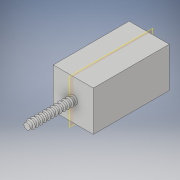
# Autodesk Inventor part: Square-Circle-Adapter V1D2-OUT
Saved by Autodesk Inventor 2017 (Build 210142000, 142)
## iProperties
Created: 2017-12-22
Part Number: Square-Circle-Adapter V1D2-OUT
Material: Generic
Document SubType Name: Modeling
Designer: Tripl_000
Density: 1 g/cm^3
Appearance: Default
Author: Tripl_000
Autodesk Inventor part; units mm, degrees
ref_plane "YZ Plane" through (0, 0, 0) normal (1, 0, 0) x (0, 1, 0)
ref_plane "XZ Plane" through (0, 0, 0) normal (0, 1, 0) x (-1, 0, 0)
ref_plane "XY Plane" through (0, 0, 0) normal (0, 0, 1) x (1, 0, 0)
sketch "Sketch1" plane through (0, 0, 0) normal (0, 0, 1) x (1, 0, 0)
  line L0 (-6.604, 6.604) -> (6.604, 6.604)
  line L1 (6.604, 6.604) -> (6.604, -6.604)
  line L2 (6.604, -6.604) -> (-6.604, -6.604)
  line L3 (-6.604, -6.604) -> (-6.604, 6.604)
  line L4 (-6.604, 6.604) -> (6.604, -6.604) construction
  line L5 (6.604, 6.604) -> (-6.604, -6.604) construction
  point P0 (0, 0)
  dimension "d0" = 13.208
  dimension "d1" = 13.208
  constraints: 12 end point, 2 midpoint, 2 parallel, 1 horizontal, 1 perpendicular
  measures "d0" distance of L2.end L0.start
  measures "d1" distance of L0.start L0.end
extrude "Extrusion1" add sketch "Sketch1" along normal blind 15
sketch "Sketch2" plane through (0, 0, 15) normal (0, 0, 1) x (1, 0, 0)
  line L0 (-5.0165, 5.0165) -> (5.0165, 5.0165)
  line L1 (5.0165, 5.0165) -> (5.0165, -5.0165)
  line L2 (5.0165, -5.0165) -> (-5.0165, -5.0165)
  line L3 (-5.0165, -5.0165) -> (-5.0165, 5.0165)
  line L4 (-5.0165, 5.0165) -> (5.0165, -5.0165) construction
  line L5 (5.0165, 5.0165) -> (-5.0165, -5.0165) construction
  point P0 (0, 0)
  dimension "d4" = 10.033
  dimension "d5" = 10.033
  constraints: 12 end point, 2 midpoint, 2 parallel, 1 horizontal, 1 perpendicular
  measures "d4" distance of L0.end L1.end
  measures "d5" distance of L0.start L0.end
extrude "Extrusion2" cut sketch "Sketch2" against normal through all
sketch "Sketch5" plane through (0, 0, 15) normal (0, 0, 1) x (1, 0, 0)
  line L0 (6.604, 6.604) -> (-6.604, 6.604) projected
  line L1 (6.604, 6.604) -> (6.604, -6.604) projected
  line L2 (-6.604, 6.604) -> (6.604, 6.604)
  line L3 (6.604, 6.604) -> (6.604, -6.604)
  line L4 (6.604, -6.604) -> (-6.604, -6.604)
  line L5 (-6.604, -6.604) -> (-6.604, 6.604)
  point P0 (0, 0)
  constraints: 8 end point, 2 parallel, 1 horizontal, 1 perpendicular
extrude "Extrusion5" add sketch "Sketch5" along normal blind 10
sketch "Sketch8" plane through (0, 0, 25) normal (0, 0, 1) x (1, 0, 0)
  circle A0 centre (0, 0) radius 0.762
  dimension "d44" = 1.524
  constraints: 1 centre point, 1 coincident
  measures "d44" diameter of A0
extrude "Extrusion7" add sketch "Sketch8" along normal blind 15.24
sketch "Sketch9" plane through (0, 0, 25) normal (0, 0, 1) x (1, 0, 0)
  circle A0 centre (0, 0) radius 1.016
  dimension "d47" = 2.032
  constraints: 1 centre point, 1 coincident
  measures "d47" diameter of A0
extrude "Extrusion8" add sketch "Sketch9" along normal up to surface (15.24 mm away)
ref_plane "Work Plane3" through (0, -6.604, 0) normal (1, 0, 0) x (0, 0, -1)
sketch "Sketch10" plane through (0, -6.604, 0) normal (1, 0, 0) x (0, 0, -1)
  line L0 (21.7384, 6.604) -> (-63.7893, 6.604)
  line L1 (-25, 5.588) -> (-25, 7.62) projected
  line L2 (-25, 7.62) -> (-25, 8.001)
  line L3 (-25, 0) -> (-25, 13.208) projected
  line L4 (-25, 8.001) -> (-25.381, 7.62)
  line L5 (-25, 7.62) -> (-40.24, 7.62) projected
  line L6 (-25.381, 7.62) -> (-25, 7.62)
  line L7 (-26.27, 7.62) -> (-26.27, 8.001)
  line L8 (-26.27, 8.001) -> (-26.651, 7.62)
  line L9 (-26.651, 7.62) -> (-26.27, 7.62)
  line L10 (-27.54, 7.62) -> (-27.54, 8.001)
  line L11 (-27.54, 8.001) -> (-27.921, 7.62)
  line L12 (-28.81, 7.62) -> (-28.81, 8.001)
  line L13 (-28.81, 8.001) -> (-29.191, 7.62)
  line L14 (-29.191, 7.62) -> (-28.81, 7.62)
  line L15 (-30.08, 7.62) -> (-30.08, 8.001)
  line L16 (-30.08, 8.001) -> (-30.461, 7.62)
  line L17 (-30.08, 7.62) -> (-30.461, 7.62)
  line L18 (-31.35, 7.62) -> (-31.35, 8.001)
  line L19 (-31.35, 8.001) -> (-31.731, 7.62)
  line L20 (-31.731, 7.62) -> (-31.35, 7.62)
  line L21 (-32.62, 7.62) -> (-32.62, 8.001)
  line L22 (-32.62, 8.001) -> (-33.001, 7.62)
  line L23 (-32.62, 7.62) -> (-33.001, 7.62)
  line L24 (-33.89, 7.62) -> (-33.89, 8.001)
  line L25 (-33.89, 8.001) -> (-34.271, 7.62)
  line L26 (-33.89, 7.62) -> (-34.271, 7.62)
  line L27 (-35.16, 7.62) -> (-35.16, 8.001)
  line L28 (-35.16, 8.001) -> (-35.541, 7.62)
  line L29 (-35.16, 7.62) -> (-35.541, 7.62)
  line L30 (-36.43, 7.62) -> (-36.43, 8.001)
  line L31 (-36.43, 8.001) -> (-36.811, 7.62)
  line L32 (-36.43, 7.62) -> (-36.811, 7.62)
  line L33 (-37.7, 7.62) -> (-37.7, 8.001)
  line L34 (-37.7, 8.001) -> (-38.081, 7.62)
  line L35 (-37.7, 7.62) -> (-38.081, 7.62)
  line L36 (-38.97, 7.62) -> (-38.97, 8.001)
  line L37 (-38.97, 8.001) -> (-39.351, 7.62)
  line L38 (-38.97, 7.62) -> (-39.351, 7.62)
  line L39 (-27.921, 7.62) -> (-27.54, 7.62)
  point P0 (0, 6.604)
  dimension "d51" = 0.381
  dimension "d52" = 45
  dimension "d53" = 0.381
  dimension "d54" = 0.381
  dimension "d55" = 0.381
  dimension "d56" = 0.381
  dimension "d57" = 0.381
  dimension "d58" = 0.381
  dimension "d59" = 0.381
  dimension "d60" = 0.381
  dimension "d61" = 0.381
  dimension "d62" = 0.381
  dimension "d63" = 0.381
  dimension "d64" = 1.27
  dimension "d65" = 1.27
  dimension "d66" = 1.27
  dimension "d67" = 1.27
  dimension "d68" = 1.27
  dimension "d69" = 1.27
  dimension "d70" = 1.27
  dimension "d71" = 1.27
  dimension "d72" = 1.27
  dimension "d73" = 1.27
  dimension "d74" = 1.27
  dimension "d75" = 0.381
  dimension "d76" = 0.381
  constraints: 74 end point, 11 vertical, 9 horizontal, 9 parallel, 4 perpendicular, 1 point on line, 23 other
  measures "d51" distance of L1.end L2.end
  measures "d52" angle of L2 L4
  measures "d53" distance of L36.start L36.end
  measures "d54" distance of L33.start L33.end
  measures "d55" distance of L30.start L30.end
  measures "d56" distance of L27.start L27.end
  measures "d57" distance of L24.start L24.end
  measures "d58" distance of L21.start L21.end
  measures "d59" distance of L18.start L18.end
  measures "d60" distance of L15.start L15.end
  measures "d61" distance of L12.start L12.end
  measures "d62" distance of L10.start L10.end
  measures "d63" distance of L7.start L7.end
  measures "d64" distance between parallel lines of L33 L36
  measures "d65" distance between parallel lines of L30 L33
  measures "d66" distance between parallel lines of L27 L30
  measures "d67" distance between parallel lines of L24 L27
  measures "d68" distance between parallel lines of L21 L24
  measures "d69" distance between parallel lines of L18 L21
  measures "d70" distance between parallel lines of L15 L18
  measures "d71" distance between parallel lines of L12 L15
  measures "d72" distance between parallel lines of L10 L12
  measures "d73" distance between parallel lines of L7 L10
  measures "d74" distance from line of L2.end L7
  measures "d75" distance of L36.start L37.end
  measures "d76" distance of L10.start L11.end
revolve "Revolution2" add sketch "Sketch10" angle 360 about axis through (0, 0, -21.7384) along (0, 0, 1)
body "Solid1"
